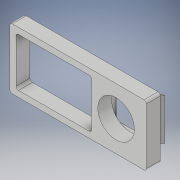
# Autodesk Inventor part: 30_Smartphone_Holder_v3
Saved by Autodesk Inventor 2019 (Build 230136000, 136)
## iProperties
Created: 2020-08-03
Part Number: 30_Smartphone_Holder_v3
Material: Generic
Document SubType Name: Modeling
Designer: marsikovabarbora
Density: 1 g/cm^3
Appearance: Default
Author: marsikovabarbora
Autodesk Inventor part; units mm, degrees
ref_plane "YZ Plane" through (0, 0, 0) normal (1, 0, 0) x (0, 1, 0)
ref_plane "XZ Plane" through (0, 0, 0) normal (0, 1, 0) x (-1, 0, 0)
ref_plane "XY Plane" through (0, 0, 0) normal (0, 0, 1) x (1, 0, 0)
sketch "Sketch1" plane through (0, 0, 0) normal (0, 0, 1) x (1, 0, 0)
  circle A0 centre (44.9, 4.9) radius 1.45 construction
  circle A1 centre (4.9, 4.9) radius 1.45 construction
  line L0 (2, 2) -> (2, 41.8) construction
  line L1 (47.8, 2) -> (2, 2) construction
  line L2 (47.8, 41.8) -> (47.8, 2) construction
  line L3 (41.8, 41.8) -> (47.8, 41.8) construction
  line L4 (41.8, 8) -> (41.8, 41.8) construction
  line L5 (8, 8) -> (41.8, 8) construction
  line L6 (8, 8) -> (8, 41.8) construction
  line L7 (2, 41.8) -> (8, 41.8) construction
  circle A2 centre (44.9, 44.9) radius 1.4 construction
  circle A3 centre (4.9, 44.9) radius 1.4 construction
  line L8 (2, 47.8) -> (47.8, 47.8) construction
  line L9 (2, 41.8) -> (2, 47.8) construction
  line L10 (47.8, 41.8) -> (2, 41.8) construction
  line L11 (47.8, 41.8) -> (47.8, 47.8) construction
  circle A4 centre (25.6838, 25.4066) radius 13.6 construction
  line L12 (44.1319, 49.8) -> (5.6681, 49.8) construction
  arc A5 (49.8, 47.8) -> (47.8, 49.8) centre (47.8, 47.8) ccw construction
  line L13 (49.8, 41.8) -> (49.8, 47.8) construction
  arc A6 (2, 49.8) -> (0, 47.8) centre (2, 47.8) ccw construction
  arc A7 (0, 2) -> (2, 0) centre (2, 2) ccw construction
  arc A8 (47.8, 0) -> (49.8, 2) centre (47.8, 2) ccw construction
  line L14 (49.8, 0) -> (-62.2, 0)
  line L15 (-62.2, 0) -> (-62.2, 49.8)
  line L16 (-62.2, 49.8) -> (49.8, 49.8)
  line L17 (49.8, 49.8) -> (49.8, 0)
  line L18 (8, 3.7577) -> (41.8, 3.7577) construction
  line L19 (41.8, 0) -> (41.8, 3.7577) construction
  line L20 (8, 0) -> (41.8, 0) construction
  line L21 (8, 0) -> (8, 3.7577) construction
  line L22 (46.1838, 8) -> (46.1838, 41.8) construction
  line L23 (49.8, 41.8) -> (46.1838, 41.8) construction
  line L24 (49.8, 8) -> (49.8, 41.8) construction
  line L25 (46.1838, 8) -> (49.8, 8) construction
  line L26 (3.6162, 41.8) -> (3.6162, 8) construction
  line L27 (0, 8) -> (3.6162, 8) construction
  line L28 (0, 8) -> (0, 41.8) construction
  line L29 (3.6162, 41.8) -> (0, 41.8) construction
  circle A9 centre (24.9, 24.9) radius 15
  arc A10 (42.3945, 24.4616) -> (22.4616, 42.2293) centre (24.9, 24.9) ccw construction
  arc A11 (22.5619, 16.1033) -> (42.3945, 24.4616) centre (29.0002, 28.5351) ccw construction
  line L30 (22.5619, 16.1033) -> (22.3031, 15.1374) construction
  arc A12 (22.3031, 15.1374) -> (41.5232, 19.4302) centre (29.3361, 28.8218) ccw construction
  arc A13 (15.3425, 10.2404) -> (41.5232, 19.4302) centre (24.9, 24.9) ccw construction
  arc A14 (18.2047, 31.6263) -> (15.3425, 10.2404) centre (25.6173, 19.7498) ccw construction
  line L31 (18.2047, 31.6263) -> (17.4976, 32.3335) construction
  arc A15 (17.4976, 32.3335) -> (11.1478, 14.0775) centre (25.6302, 19.2725) ccw construction
  arc A16 (16.2809, 40.1303) -> (11.1478, 14.0775) centre (24.9, 24.9) ccw construction
  arc A17 (34.0602, 27.4798) -> (16.2809, 40.1303) centre (20.0844, 26.6568) ccw construction
  line L32 (34.0602, 27.4798) -> (35.0261, 27.7386) construction
  arc A18 (35.0261, 27.7386) -> (22.4616, 42.2293) centre (19.6533, 27.1018) ccw construction
  line L33 (3.6577, 41.7) -> (8.1, 46.1423) construction
  line L34 (0, 41.7) -> (3.6577, 41.7) construction
  line L35 (0, 8.1) -> (0, 41.7) construction
  line L36 (3.6577, 8.1) -> (0, 8.1) construction
  line L37 (8.1, 3.6577) -> (3.6577, 8.1) construction
  line L38 (8.1, 0) -> (8.1, 3.6577) construction
  line L39 (41.7, 0) -> (8.1, 0) construction
  line L40 (41.7, 3.6577) -> (41.7, 0) construction
  line L41 (46.1423, 8.1) -> (41.7, 3.6577) construction
  line L42 (49.8, 8.1) -> (46.1423, 8.1) construction
  line L43 (49.8, 41.7) -> (49.8, 8.1) construction
  line L44 (46.1423, 41.7) -> (49.8, 41.7) construction
  line L45 (41.7, 46.1423) -> (46.1423, 41.7) construction
  line L46 (41.7, 49.8) -> (41.7, 46.1423) construction
  line L47 (8.1, 49.8) -> (41.7, 49.8) construction
  line L48 (8.1, 46.1423) -> (8.1, 49.8) construction
  circle A19 centre (24.9, 24.9) radius 16.9 construction
  point P0 (0, 0)
  dimension "d0" = 30
  dimension "d4" = 112
  constraints: 8 end point, 3 collinear, 2 parallel, 1 centre point, 1 coincident, 1 horizontal, 1 perpendicular
  measures "d0" diameter of A9
  measures "d4" distance between parallel lines of L43 L15
extrude "Extrusion1" add sketch "Sketch1" along normal blind 11.4
fillet "Fillet1" radius 2 4 edges at (49.8, 49.8, 5.7) (-62.2, 49.8, 5.7) (49.8, 0, 5.7) (-62.2, 0, 5.7)
sketch "Sketch2" plane through (0, 0, 0) normal (0, 0, -1) x (-1, 0, 0)
  line L0 (-41.8, 8) -> (-41.8, 41.8) construction
  line L1 (-8, 8) -> (-41.8, 8) construction
  line L2 (-8, 8) -> (-8, 41.8) construction
  line L3 (-47.8, 41.8) -> (-2, 41.8) construction
  circle A0 centre (-24.9, 24.9) radius 15 construction
  arc A1 (60.2, 0) -> (62.2, 2) centre (60.2, 2) ccw construction
  line L4 (62.2, 2) -> (62.2, 47.8) construction
  arc A2 (62.2, 47.8) -> (60.2, 49.8) centre (60.2, 47.8) ccw construction
  line L5 (60.2, 49.8) -> (-47.8, 49.8) construction
  arc A3 (-47.8, 49.8) -> (-49.8, 47.8) centre (-47.8, 47.8) ccw construction
  line L6 (-49.8, 47.8) -> (-49.8, 2) construction
  arc A4 (-49.8, 2) -> (-47.8, 0) centre (-47.8, 2) ccw construction
  line L7 (-47.8, 0) -> (60.2, 0) construction
  line L8 (-41.8, 41.8) -> (-8, 41.8)
  line L9 (-8, 41.8) -> (-8, 8)
  line L10 (-8, 8) -> (-41.8, 8)
  line L11 (-41.8, 8) -> (-41.8, 41.8)
  line L12 (-9, 40.8) -> (-40.8, 40.8)
  line L13 (-40.8, 40.8) -> (-40.8, 9)
  line L14 (-40.8, 9) -> (-9, 9)
  line L15 (-9, 9) -> (-9, 40.8)
  point P0 (0, 0)
  dimension "d6" = 0
  dimension "d7" = 0
  dimension "d8" = 0
  dimension "d9" = 0
  dimension "d10" = 1
  constraints: 16 end point, 4 parallel, 2 perpendicular, 1 horizontal, 3 other
  measures "d6" distance between parallel lines of L3 L8
  measures "d7" distance between parallel lines of L0 L11
  measures "d8" distance between parallel lines of L2 L9
  measures "d9" distance between parallel lines of L1 L10
  measures "d10" distance between parallel lines of L8 L12
extrude "Extrusion2" add sketch "Sketch2" along normal blind 3.66
sketch "Sketch3" plane through (8, 8, 0) normal (0, -1, 0) x (1, 0, 0)
  line L0 (0, 0) -> (33.8, 0) construction
  line L1 (0, 0) -> (0, -3.66) construction
  line L2 (33.8, -3.66) -> (0, -3.66) construction
  line L3 (33.8, 0) -> (33.8, -3.66) construction
  line L4 (33.5, -3.7577) -> (33.5, -8) construction
  line L5 (-0.3, -8) -> (33.5, -8) construction
  line L6 (-0.3, -3.7577) -> (-0.3, -8) construction
  line L7 (33.5, -3.7577) -> (-0.3, -3.7577) construction
  line L8 (33.5, 0) -> (33.5, -3.6162) construction
  line L9 (-0.3, -3.6162) -> (-0.3, 0) construction
  line L10 (33.8, 0) -> (33.8, -3.66) construction
  line L11 (33.8, 0) -> (33.8, -3.66) construction
  line L12 (33.5, -8) -> (33.5, -3.7577) construction
  line L13 (33.5, -3.7577) -> (-0.3, -3.7577) construction
  line L14 (-0.3, -3.7577) -> (-0.3, -8) construction
  line L15 (-0.3, -8) -> (-4.6838, -8) construction
  line L16 (-2.886, -6.2022) -> (-4.6838, -8) construction
  arc A0 (-2.886, -6.2022) -> (-2.0978, -5.414) centre (-3.4, -4.9) ccw construction
  line L17 (-0.3, -3.6162) -> (-2.0978, -5.414) construction
  line L18 (-0.3, -3.6162) -> (-0.3, 0) construction
  line L19 (-0.3, 0) -> (33.5, 0) construction
  line L20 (33.5, 0) -> (33.5, -3.6162) construction
  line L21 (35.2978, -5.414) -> (33.5, -3.6162) construction
  arc A1 (35.2978, -5.414) -> (36.086, -6.2022) centre (36.6, -4.9) ccw construction
  line L22 (37.8838, -8) -> (36.086, -6.2022) construction
  line L23 (37.8838, -8) -> (33.5, -8) construction
  line L24 (0, -3.66) -> (33.8, -3.66) projected
  line L25 (0, -3.66) -> (-4.34, -8)
  line L26 (-4.34, -8) -> (-2.2187, -8)
  line L27 (-2.2187, -8) -> (2.1213, -3.66)
  line L28 (16.6, -3.7577) -> (16.6, -8) construction
  line L29 (2.1213, -3.66) -> (0, -3.66)
  line L30 (1, -3.66) -> (32.8, -3.66) projected
  line L31 (33.5, -3.7577) -> (33.5, -8) construction
  line L32 (33.5, -3.7577) -> (33.5, -8) construction
  line L33 (33.5, -8) -> (37.8838, -8) construction
  line L34 (36.086, -6.2022) -> (37.8838, -8) construction
  arc A2 (35.2978, -5.414) -> (36.086, -6.2022) centre (36.6, -4.9) ccw construction
  line L35 (33.5, -3.6162) -> (35.2978, -5.414) construction
  line L36 (33.2, -3.66) -> (37.54, -8)
  line L37 (37.54, -8) -> (35.4187, -8)
  line L38 (35.4187, -8) -> (31.0787, -3.66)
  line L39 (31.0787, -3.66) -> (33.2, -3.66)
  point P0 (-8, 0)
  point P1 (32.2, -3.66)
  dimension "d13" = 1.5
  constraints: 28 end point, 6 symmetric about line, 5 point on line, 2 midpoint, 2 parallel, 2 point on circle, 1 centre point, 1 collinear, 1 other
  measures "d13" distance between parallel lines of L27 L25
extrude "Extrusion3" add sketch "Sketch3" against normal up to surface (33.8 mm away)
sketch "Sketch4" plane through (0, 0, 0) normal (0, 0, -1) x (-1, 0, 0)
  arc A0 (60.2, 0) -> (62.2, 2) centre (60.2, 2) ccw construction
  line L0 (62.2, 2) -> (62.2, 47.8) construction
  arc A1 (62.2, 47.8) -> (60.2, 49.8) centre (60.2, 47.8) ccw construction
  line L1 (60.2, 49.8) -> (-47.8, 49.8) construction
  arc A2 (-47.8, 49.8) -> (-49.8, 47.8) centre (-47.8, 47.8) ccw construction
  line L2 (-49.8, 47.8) -> (-49.8, 2) construction
  arc A3 (-49.8, 2) -> (-47.8, 0) centre (-47.8, 2) ccw construction
  line L3 (-47.8, 0) -> (60.2, 0) construction
  line L4 (-8, 41.8) -> (-8, 8) construction
  line L5 (-8, 8) -> (-41.8, 8) construction
  line L6 (-41.8, 8) -> (-41.8, 41.8) construction
  line L7 (-41.8, 41.8) -> (-8, 41.8) construction
  line L8 (-4.8, 44.8) -> (57.2, 44.8)
  line L9 (57.2, 44.8) -> (57.2, 5)
  line L10 (57.2, 5) -> (-4.8, 5)
  line L11 (-4.8, 5) -> (-4.8, 44.8)
  point P0 (0, 0)
  dimension "d16" = 45
  dimension "d17" = 5
  dimension "d18" = 5
  dimension "d19" = 5
  constraints: 8 end point, 2 parallel, 1 horizontal, 1 perpendicular
  measures "d16" distance between parallel lines of L11 L2
  measures "d17" distance between parallel lines of L1 L8
  measures "d18" distance between parallel lines of L3 L10
  measures "d19" distance between parallel lines of L0 L9
extrude "Extrusion4" cut sketch "Sketch4" against normal through all
fillet "Fillet2" radius 2 4 edges at (4.8, 5, 5.7) (-57.2, 5, 5.7) (-57.2, 44.8, 5.7) (4.8, 44.8, 5.7)
equation "\"d18\" = d17"
equation "\"d19\" = d17"
body "Solid1"
